Autodesk Inventor part; units mm, degrees
(part 7 of 8)
  arc A913 (19.6836, 30.4546) -> (19.6836, 30.4038) centre (19.6836, 30.4292) ccw
  arc A914 (19.9605, 30.3115) -> (19.991, 30.3522) centre (19.9757, 30.3318) ccw
  arc A915 (19.9757, 30.3318) -> (19.6836, 30.4292) centre (19.6836, 29.9424) ccw
  arc A916 (19.3986, 30.1696) -> (19.4494, 30.1696) centre (19.424, 30.1696) ccw
  arc A917 (19.6836, 30.4038) -> (19.6836, 30.4546) centre (19.6836, 30.4292) ccw
  arc A918 (19.6836, 30.4292) -> (19.424, 30.1696) centre (19.6836, 30.1696) ccw
  arc A919 (19.781, 29.2354) -> (19.781, 29.2862) centre (19.781, 29.2608) ccw
  arc A920 (19.4096, 29.441) -> (19.3735, 29.4052) centre (19.3916, 29.4231) ccw
  arc A921 (19.3915, 29.4231) -> (19.781, 29.2608) centre (19.781, 29.8093) ccw
  arc A922 (20.066, 29.5204) -> (20.0152, 29.5204) centre (20.0406, 29.5204) ccw
  arc A923 (19.781, 29.2862) -> (19.781, 29.2354) centre (19.781, 29.2608) ccw
  arc A924 (19.781, 29.2608) -> (20.0406, 29.5204) centre (19.781, 29.5204) ccw
  arc A925 (18.9204, 29.2494) -> (18.9658, 29.2722) centre (18.9431, 29.2608) ccw
  arc A926 (18.7062, 29.7914) -> (18.6607, 29.7687) centre (18.6835, 29.78) ccw
  line L282 (18.9431, 29.2608) -> (18.6835, 29.7801)
  arc A927 (18.6185, 29.7547) -> (18.6185, 29.8055) centre (18.6185, 29.7801) ccw
  arc A928 (18.294, 29.8055) -> (18.294, 29.7547) centre (18.294, 29.7801) ccw
  line L283 (18.6185, 29.7801) -> (18.294, 29.7801)
  arc A929 (18.6185, 30.4546) -> (18.6185, 30.4038) centre (18.6185, 30.4292) ccw
  arc A930 (18.6185, 29.8055) -> (18.6185, 29.7547) centre (18.6185, 29.7801) ccw
  arc A931 (18.6185, 29.7801) -> (18.6185, 30.4292) centre (18.6185, 30.1046) ccw
  arc A932 (18.294, 30.4546) -> (18.294, 30.4038) centre (18.294, 30.4292) ccw
  arc A933 (18.6185, 30.4038) -> (18.6185, 30.4546) centre (18.6185, 30.4292) ccw
  line L284 (18.294, 30.4292) -> (18.6185, 30.4292)
  arc A934 (18.2686, 29.2608) -> (18.3194, 29.2608) centre (18.294, 29.2608) ccw
  arc A935 (18.3194, 30.4292) -> (18.2686, 30.4292) centre (18.294, 30.4292) ccw
  line L285 (18.294, 29.2608) -> (18.294, 30.4292)
  arc A936 (17.78, 29.5854) -> (17.7292, 29.5854) centre (17.7546, 29.5854) ccw
  arc A937 (17.1309, 29.5854) -> (17.0801, 29.5854) centre (17.1055, 29.5854) ccw
  arc A938 (17.1055, 29.5854) -> (17.7546, 29.5854) centre (17.4301, 29.5854) ccw
  arc A939 (17.78, 30.1046) -> (17.7292, 30.1046) centre (17.7546, 30.1046) ccw
  arc A940 (17.7292, 29.5854) -> (17.78, 29.5854) centre (17.7546, 29.5854) ccw
  line L286 (17.7546, 30.1046) -> (17.7546, 29.5854)
  arc A941 (17.0801, 30.1046) -> (17.1309, 30.1046) centre (17.1055, 30.1046) ccw
  arc A942 (17.7292, 30.1046) -> (17.78, 30.1046) centre (17.7546, 30.1046) ccw
  arc A943 (17.7546, 30.1046) -> (17.1055, 30.1046) centre (17.4301, 30.1046) ccw
  arc A944 (17.0801, 29.5854) -> (17.1309, 29.5854) centre (17.1055, 29.5854) ccw
  arc A945 (17.1309, 30.1046) -> (17.0801, 30.1046) centre (17.1055, 30.1046) ccw
  line L287 (17.1055, 29.5854) -> (17.1055, 30.1046)
  arc A946 (16.5078, 29.7253) -> (16.5321, 29.7699) centre (16.5199, 29.7476) ccw
  arc A947 (16.1751, 29.9647) -> (16.1507, 29.9201) centre (16.1629, 29.9424) ccw
  line L288 (16.5199, 29.7476) -> (16.1629, 29.9424)
  arc A948 (16.5328, 29.7695) -> (16.507, 29.7257) centre (16.5199, 29.7476) ccw
  arc A949 (16.6243, 29.5204) -> (16.6751, 29.5204) centre (16.6497, 29.5204) ccw
  arc A950 (16.6497, 29.5204) -> (16.5199, 29.7476) centre (16.3861, 29.5204) ccw
  arc A951 (16.15, 29.9205) -> (16.1758, 29.9642) centre (16.1629, 29.9424) ccw
  arc A952 (16.0585, 30.1696) -> (16.0077, 30.1696) centre (16.0331, 30.1696) ccw
  arc A953 (16.0331, 30.1696) -> (16.1629, 29.9424) centre (16.2968, 30.1695) ccw
  arc A954 (16.2927, 30.4546) -> (16.2927, 30.4038) centre (16.2927, 30.4292) ccw
  arc A955 (16.5696, 30.3115) -> (16.6001, 30.3522) centre (16.5849, 30.3318) ccw
  arc A956 (16.5848, 30.3318) -> (16.2927, 30.4292) centre (16.2927, 29.9424) ccw
  arc A957 (16.0077, 30.1696) -> (16.0585, 30.1696) centre (16.0331, 30.1696) ccw
  arc A958 (16.2927, 30.4038) -> (16.2927, 30.4546) centre (16.2927, 30.4292) ccw
  arc A959 (16.2927, 30.4292) -> (16.0331, 30.1696) centre (16.2927, 30.1696) ccw
  arc A960 (16.3901, 29.2354) -> (16.3901, 29.2862) centre (16.3901, 29.2608) ccw
  arc A961 (16.0187, 29.441) -> (15.9826, 29.4052) centre (16.0007, 29.4231) ccw
  arc A962 (16.0006, 29.4231) -> (16.3901, 29.2608) centre (16.3901, 29.8093) ccw
  arc A963 (16.6751, 29.5204) -> (16.6243, 29.5204) centre (16.6497, 29.5204) ccw
  arc A964 (16.3901, 29.2862) -> (16.3901, 29.2354) centre (16.3901, 29.2608) ccw
  arc A965 (16.3901, 29.2608) -> (16.6497, 29.5204) centre (16.3901, 29.5204) ccw
  arc A966 (15.4813, 29.2608) -> (15.5321, 29.2608) centre (15.5067, 29.2608) ccw
  arc A967 (15.5321, 30.4292) -> (15.4813, 30.4292) centre (15.5067, 30.4292) ccw
  line L289 (15.5067, 29.2608) -> (15.5067, 30.4292)
  arc A968 (14.8798, 30.4415) -> (14.8354, 30.4169) centre (14.8576, 30.4292) ccw
  arc A969 (15.4845, 29.2485) -> (15.5289, 29.2731) centre (15.5067, 29.2608) ccw
  line L290 (14.8576, 30.4292) -> (15.5067, 29.2608)
  arc A970 (14.8322, 29.2608) -> (14.883, 29.2608) centre (14.8576, 29.2608) ccw
  arc A971 (14.883, 30.4292) -> (14.8322, 30.4292) centre (14.8576, 30.4292) ccw
  line L291 (14.8576, 29.2608) -> (14.8576, 30.4292)
  arc A972 (13.8693, 29.9353) -> (13.8693, 29.8845) centre (13.8693, 29.9099) ccw
  arc A973 (14.2588, 29.8845) -> (14.2588, 29.9353) centre (14.2588, 29.9099) ccw
  line L292 (13.8693, 29.9099) -> (14.2588, 29.9099)
  arc A974 (13.8693, 30.4546) -> (13.8693, 30.4038) centre (13.8693, 30.4292) ccw
  arc A975 (14.3886, 30.4038) -> (14.3886, 30.4546) centre (14.3886, 30.4292) ccw
  line L293 (13.8693, 30.4292) -> (14.3886, 30.4292)
  arc A976 (13.8439, 29.2608) -> (13.8947, 29.2608) centre (13.8693, 29.2608) ccw
  arc A977 (13.8947, 30.4292) -> (13.8439, 30.4292) centre (13.8693, 30.4292) ccw
  line L294 (13.8693, 29.2608) -> (13.8693, 30.4292)
  arc A978 (14.3886, 29.2354) -> (14.3886, 29.2862) centre (14.3886, 29.2608) ccw
  arc A979 (13.8693, 29.2862) -> (13.8693, 29.2354) centre (13.8693, 29.2608) ccw
  line L295 (14.3886, 29.2608) -> (13.8693, 29.2608)
  arc A980 (13.2312, 29.7253) -> (13.2555, 29.7699) centre (13.2433, 29.7476) ccw
  arc A981 (12.8985, 29.9647) -> (12.8741, 29.9201) centre (12.8863, 29.9424) ccw
  line L296 (13.2433, 29.7476) -> (12.8863, 29.9424)
  arc A982 (13.2562, 29.7695) -> (13.2304, 29.7257) centre (13.2433, 29.7476) ccw
  arc A983 (13.3477, 29.5204) -> (13.3985, 29.5204) centre (13.3731, 29.5204) ccw
  arc A984 (13.3731, 29.5204) -> (13.2433, 29.7476) centre (13.1095, 29.5204) ccw
  arc A985 (12.8734, 29.9205) -> (12.8992, 29.9642) centre (12.8863, 29.9424) ccw
  arc A986 (12.7819, 30.1696) -> (12.7311, 30.1696) centre (12.7565, 30.1696) ccw
  arc A987 (12.7565, 30.1696) -> (12.8863, 29.9424) centre (13.0202, 30.1695) ccw
  arc A988 (13.0161, 30.4546) -> (13.0161, 30.4038) centre (13.0161, 30.4292) ccw
  arc A989 (13.293, 30.3115) -> (13.3235, 30.3522) centre (13.3082, 30.3318) ccw
  arc A990 (13.3082, 30.3318) -> (13.0161, 30.4292) centre (13.0161, 29.9424) ccw
  arc A991 (12.7311, 30.1696) -> (12.7819, 30.1696) centre (12.7565, 30.1696) ccw
  arc A992 (13.0161, 30.4038) -> (13.0161, 30.4546) centre (13.0161, 30.4292) ccw
  arc A993 (13.0161, 30.4292) -> (12.7565, 30.1696) centre (13.0161, 30.1696) ccw
  arc A994 (13.1135, 29.2354) -> (13.1135, 29.2862) centre (13.1135, 29.2608) ccw
  arc A995 (12.7421, 29.441) -> (12.706, 29.4052) centre (12.7241, 29.4231) ccw
  arc A996 (12.724, 29.4231) -> (13.1135, 29.2608) centre (13.1135, 29.8093) ccw
  arc A997 (13.3985, 29.5204) -> (13.3477, 29.5204) centre (13.3731, 29.5204) ccw
  arc A998 (13.1135, 29.2862) -> (13.1135, 29.2354) centre (13.1135, 29.2608) ccw
  arc A999 (13.1135, 29.2608) -> (13.3731, 29.5204) centre (13.1135, 29.5204) ccw
  arc A1000 (83.7121, 29.1084) -> (83.801, 29.1084) centre (83.7565, 29.1084) ccw
  arc A1001 (83.801, 30.7086) -> (83.7121, 30.7086) centre (83.7566, 30.7086) ccw
  line L297 (83.7565, 29.1084) -> (83.7565, 30.7086)
  arc A1002 (82.9064, 30.7302) -> (82.8286, 30.687) centre (82.8675, 30.7086) ccw
  arc A1003 (83.7176, 29.0868) -> (83.7954, 29.13) centre (83.7565, 29.1084) ccw
  line L298 (82.8675, 30.7086) -> (83.7565, 29.1084)
  arc A1004 (82.8231, 29.1084) -> (82.912, 29.1084) centre (82.8675, 29.1084) ccw
  arc A1005 (82.912, 30.7086) -> (82.8231, 30.7086) centre (82.8676, 30.7086) ccw
  line L299 (82.8675, 29.1084) -> (82.8675, 30.7086)
  arc A1006 (81.8316, 30.7531) -> (81.8316, 30.6641) centre (81.8316, 30.7086) ccw
  arc A1007 (82.1872, 30.6641) -> (82.1872, 30.7531) centre (82.1872, 30.7086) ccw
  line L300 (81.8316, 30.7086) -> (82.1872, 30.7086)
  arc A1008 (81.8316, 29.1529) -> (81.8316, 29.064) centre (81.8316, 29.1085) ccw
  arc A1009 (82.1872, 29.064) -> (82.1872, 29.1529) centre (82.1872, 29.1085) ccw
  line L301 (81.8316, 29.1084) -> (82.1872, 29.1084)
  arc A1010 (82.0538, 30.7086) -> (81.965, 30.7086) centre (82.0094, 30.7086) ccw
  arc A1011 (81.965, 29.1084) -> (82.0538, 29.1084) centre (82.0094, 29.1084) ccw
  line L302 (82.0094, 30.7086) -> (82.0094, 29.1084)
  arc A1012 (80.5596, 28.9751) -> (80.5596, 28.8862) centre (80.5596, 28.9306) ccw
  arc A1013 (81.2708, 28.8862) -> (81.2708, 28.9751) centre (81.2708, 28.9306) ccw
  line L303 (80.5596, 28.9306) -> (81.2708, 28.9306)
  arc A1014 (79.9232, 29.0885) -> (80.0028, 29.1283) centre (79.963, 29.1084) ccw
  arc A1015 (79.6472, 29.8395) -> (79.5676, 29.7997) centre (79.6074, 29.8196) ccw
  line L304 (79.963, 29.1084) -> (79.6074, 29.8196)
  arc A1016 (79.5185, 29.7752) -> (79.5185, 29.8641) centre (79.5185, 29.8197) ccw
  arc A1017 (79.074, 29.8641) -> (79.074, 29.7752) centre (79.074, 29.8197) ccw
  line L305 (79.5185, 29.8196) -> (79.074, 29.8196)
  arc A1018 (79.5185, 30.7531) -> (79.5185, 30.6641) centre (79.5185, 30.7086) ccw
  arc A1019 (79.5185, 29.8641) -> (79.5185, 29.7752) centre (79.5185, 29.8197) ccw
  arc A1020 (79.5185, 29.8196) -> (79.5185, 30.7086) centre (79.5185, 30.2641) ccw
  arc A1021 (79.074, 30.7531) -> (79.074, 30.6641) centre (79.074, 30.7086) ccw
  arc A1022 (79.5185, 30.6641) -> (79.5185, 30.7531) centre (79.5185, 30.7086) ccw
  line L306 (79.074, 30.7086) -> (79.5185, 30.7086)
  arc A1023 (79.0295, 29.1084) -> (79.1184, 29.1084) centre (79.0739, 29.1084) ccw
  arc A1024 (79.1184, 30.7086) -> (79.0295, 30.7086) centre (79.0739, 30.7086) ccw
  line L307 (79.074, 29.1084) -> (79.074, 30.7086)
  arc A1025 (77.7125, 30.0419) -> (77.7125, 29.953) centre (77.7125, 29.9975) ccw
  arc A1026 (78.2459, 29.953) -> (78.2459, 30.0419) centre (78.2459, 29.9975) ccw
  line L308 (77.7125, 29.9974) -> (78.2459, 29.9974)
  arc A1027 (77.7125, 30.7531) -> (77.7125, 30.6641) centre (77.7125, 30.7086) ccw
  arc A1028 (78.4237, 30.6641) -> (78.4237, 30.7531) centre (78.4237, 30.7086) ccw
  line L309 (77.7125, 30.7086) -> (78.4237, 30.7086)
  arc A1029 (77.668, 29.1084) -> (77.7569, 29.1084) centre (77.7125, 29.1084) ccw
  arc A1030 (77.7569, 30.7086) -> (77.668, 30.7086) centre (77.7125, 30.7086) ccw
  line L310 (77.7125, 29.1084) -> (77.7125, 30.7086)
  arc A1031 (78.4237, 29.064) -> (78.4237, 29.1529) centre (78.4237, 29.1085) ccw
  arc A1032 (77.7125, 29.1529) -> (77.7125, 29.064) centre (77.7125, 29.1085) ccw
  line L311 (78.4237, 29.1084) -> (77.7125, 29.1084)
  arc A1033 (76.6423, 29.118) -> (76.7291, 29.0988) centre (76.6857, 29.1084) ccw
  arc A1034 (77.0847, 30.699) -> (76.9979, 30.7182) centre (77.0413, 30.7086) ccw
  line L312 (76.6857, 29.1084) -> (77.0413, 30.7086)
  arc A1035 (76.3722, 30.1893) -> (76.2879, 30.1611) centre (76.33, 30.1752) ccw
  arc A1036 (76.6435, 29.0943) -> (76.7278, 29.1225) centre (76.6857, 29.1084) ccw
  line L313 (76.3301, 30.1752) -> (76.6857, 29.1084)
  arc A1037 (75.9323, 29.1225) -> (76.0166, 29.0943) centre (75.9744, 29.1084) ccw
  arc A1038 (76.3722, 30.1611) -> (76.2879, 30.1893) centre (76.33, 30.1752) ccw
  line L314 (75.9745, 29.1084) -> (76.3301, 30.1752)
  arc A1039 (75.6623, 30.7182) -> (75.5755, 30.699) centre (75.6189, 30.7086) ccw
  arc A1040 (75.9311, 29.0988) -> (76.0179, 29.118) centre (75.9745, 29.1084) ccw
  line L315 (75.6189, 30.7086) -> (75.9745, 29.1084)
  arc A1041 (75.0475, 29.5529) -> (74.9586, 29.5529) centre (75.0031, 29.5529) ccw
  arc A1042 (74.1585, 29.5529) -> (74.0696, 29.5529) centre (74.114, 29.5529) ccw
  arc A1043 (74.114, 29.5529) -> (75.003, 29.5529) centre (74.5585, 29.5529) ccw
  arc A1044 (75.0475, 30.2641) -> (74.9586, 30.2641) centre (75.0031, 30.2641) ccw
  arc A1045 (74.9586, 29.5529) -> (75.0475, 29.5529) centre (75.0031, 29.5529) ccw
  line L316 (75.003, 30.2641) -> (75.003, 29.5529)
  arc A1046 (74.0696, 30.2641) -> (74.1585, 30.2641) centre (74.114, 30.2641) ccw
  arc A1047 (74.9586, 30.2641) -> (75.0475, 30.2641) centre (75.0031, 30.2641) ccw
  arc A1048 (75.003, 30.2641) -> (74.114, 30.2641) centre (74.5585, 30.2641) ccw
  arc A1049 (74.0696, 29.5529) -> (74.1585, 29.5529) centre (74.114, 29.5529) ccw
  arc A1050 (74.1585, 30.2641) -> (74.0696, 30.2641) centre (74.114, 30.2641) ccw
  line L317 (74.114, 29.5529) -> (74.114, 30.2641)
  arc A1051 (73.0707, 29.7752) -> (73.0707, 29.8641) centre (73.0707, 29.8197) ccw
  arc A1052 (72.6262, 29.8641) -> (72.6262, 29.7752) centre (72.6262, 29.8197) ccw
  line L318 (73.0707, 29.8196) -> (72.6262, 29.8196)
  arc A1053 (73.0707, 30.7531) -> (73.0707, 30.6641) centre (73.0707, 30.7086) ccw
  arc A1054 (73.0707, 29.8641) -> (73.0707, 29.7752) centre (73.0707, 29.8197) ccw
  arc A1055 (73.0707, 29.8196) -> (73.0707, 30.7086) centre (73.0707, 30.2641) ccw
  arc A1056 (72.6262, 30.7531) -> (72.6262, 30.6641) centre (72.6262, 30.7086) ccw
  arc A1057 (73.0707, 30.6641) -> (73.0707, 30.7531) centre (73.0707, 30.7086) ccw
  line L319 (72.6262, 30.7086) -> (73.0707, 30.7086)
  arc A1058 (72.5818, 29.1084) -> (72.6707, 29.1084) centre (72.6262, 29.1084) ccw
  arc A1059 (72.6707, 30.7086) -> (72.5818, 30.7086) centre (72.6262, 30.7086) ccw
  line L320 (72.6262, 29.1084) -> (72.6262, 30.7086)
  arc A1060 (59.8236, 29.7253) -> (59.8479, 29.7699) centre (59.8358, 29.7476) ccw
  arc A1061 (59.4909, 29.9647) -> (59.4666, 29.9201) centre (59.4788, 29.9424) ccw
  line L321 (59.8358, 29.7476) -> (59.4788, 29.9424)
  arc A1062 (59.8487, 29.7695) -> (59.8229, 29.7257) centre (59.8358, 29.7476) ccw
  arc A1063 (59.9402, 29.5204) -> (59.991, 29.5204) centre (59.9656, 29.5204) ccw
  arc A1064 (59.9656, 29.5204) -> (59.8358, 29.7476) centre (59.7019, 29.5204) ccw
  arc A1065 (59.4659, 29.9205) -> (59.4916, 29.9642) centre (59.4787, 29.9424) ccw
  arc A1066 (59.3743, 30.1696) -> (59.3235, 30.1696) centre (59.3489, 30.1696) ccw
  arc A1067 (59.3489, 30.1696) -> (59.4788, 29.9424) centre (59.6126, 30.1696) ccw
  arc A1068 (59.6086, 30.4546) -> (59.6086, 30.4038) centre (59.6086, 30.4292) ccw
  arc A1069 (59.8855, 30.3115) -> (59.9159, 30.3522) centre (59.9007, 30.3318) ccw
  arc A1070 (59.9007, 30.3318) -> (59.6086, 30.4292) centre (59.6086, 29.9424) ccw
  arc A1071 (59.3235, 30.1696) -> (59.3743, 30.1696) centre (59.3489, 30.1696) ccw
  arc A1072 (59.6086, 30.4038) -> (59.6086, 30.4546) centre (59.6086, 30.4292) ccw
  arc A1073 (59.6086, 30.4292) -> (59.3489, 30.1696) centre (59.6086, 30.1695) ccw
  arc A1074 (59.706, 29.2354) -> (59.706, 29.2862) centre (59.706, 29.2608) ccw
  arc A1075 (59.3345, 29.441) -> (59.2985, 29.4052) centre (59.3165, 29.4231) ccw
  arc A1076 (59.3165, 29.4231) -> (59.706, 29.2608) centre (59.706, 29.8094) ccw
  arc A1077 (59.991, 29.5204) -> (59.9402, 29.5204) centre (59.9656, 29.5204) ccw
  arc A1078 (59.706, 29.2862) -> (59.706, 29.2354) centre (59.706, 29.2608) ccw
  arc A1079 (59.706, 29.2608) -> (59.9656, 29.5204) centre (59.706, 29.5204) ccw
  arc A1080 (58.8453, 29.2494) -> (58.8908, 29.2722) centre (58.868, 29.2608) ccw
  arc A1081 (58.6311, 29.7914) -> (58.5857, 29.7687) centre (58.6084, 29.78) ccw
  line L322 (58.8681, 29.2608) -> (58.6084, 29.7801)
  arc A1082 (58.5435, 29.7547) -> (58.5435, 29.8055) centre (58.5435, 29.7801) ccw
  arc A1083 (58.219, 29.8055) -> (58.219, 29.7547) centre (58.219, 29.7801) ccw
  line L323 (58.5435, 29.7801) -> (58.219, 29.7801)
  arc A1084 (58.5435, 30.4546) -> (58.5435, 30.4038) centre (58.5435, 30.4292) ccw
  arc A1085 (58.5435, 29.8055) -> (58.5435, 29.7547) centre (58.5435, 29.7801) ccw
  arc A1086 (58.5435, 29.7801) -> (58.5435, 30.4292) centre (58.5435, 30.1046) ccw
  arc A1087 (58.5435, 30.4038) -> (58.5435, 30.4546) centre (58.5435, 30.4292) ccw
  line L324 (58.219, 30.4292) -> (58.5435, 30.4292)
  arc A1088 (58.1936, 29.2608) -> (58.2444, 29.2608) centre (58.219, 29.2608) ccw
  arc A1089 (58.2444, 30.4292) -> (58.1936, 30.4292) centre (58.219, 30.4292) ccw
  line L325 (58.219, 29.2608) -> (58.219, 30.4292)
  arc A1090 (57.705, 29.5854) -> (57.6542, 29.5854) centre (57.6796, 29.5854) ccw
  arc A1091 (57.0559, 29.5854) -> (57.0051, 29.5854) centre (57.0305, 29.5854) ccw
  arc A1092 (57.0305, 29.5854) -> (57.6796, 29.5854) centre (57.3551, 29.5854) ccw
  arc A1093 (57.705, 30.1046) -> (57.6542, 30.1046) centre (57.6796, 30.1046) ccw
  arc A1094 (57.6542, 29.5854) -> (57.705, 29.5854) centre (57.6796, 29.5854) ccw
  line L326 (57.6796, 30.1046) -> (57.6796, 29.5854)
  arc A1095 (57.0051, 30.1046) -> (57.0559, 30.1046) centre (57.0305, 30.1046) ccw
  arc A1096 (57.6542, 30.1046) -> (57.705, 30.1046) centre (57.6796, 30.1046) ccw
  arc A1097 (57.6796, 30.1046) -> (57.0305, 30.1046) centre (57.3551, 30.1046) ccw
  arc A1098 (57.0051, 29.5854) -> (57.0559, 29.5854) centre (57.0305, 29.5854) ccw
  arc A1099 (57.0559, 30.1046) -> (57.0051, 30.1046) centre (57.0305, 30.1046) ccw
  line L327 (57.0305, 29.5854) -> (57.0305, 30.1046)
  arc A1100 (55.9637, 30.4546) -> (55.9637, 30.4038) centre (55.9637, 30.4292) ccw
  arc A1101 (56.6128, 30.4038) -> (56.6128, 30.4546) centre (56.6128, 30.4292) ccw
  line L328 (55.9637, 30.4292) -> (56.6128, 30.4292)
  arc A1102 (56.2629, 29.2608) -> (56.3137, 29.2608) centre (56.2883, 29.2608) ccw
  arc A1103 (56.3137, 30.4292) -> (56.2629, 30.4292) centre (56.2883, 30.4292) ccw
  line L329 (56.2883, 29.2608) -> (56.2883, 30.4292)
  arc A1104 (55.5714, 29.5854) -> (55.5206, 29.5854) centre (55.546, 29.5854) ccw
  arc A1105 (54.9223, 29.5854) -> (54.8715, 29.5854) centre (54.8969, 29.5854) ccw
  arc A1106 (54.8969, 29.5854) -> (55.546, 29.5854) centre (55.2215, 29.5854) ccw
  arc A1107 (55.5714, 30.1046) -> (55.5206, 30.1046) centre (55.546, 30.1046) ccw
  arc A1108 (55.5206, 29.5854) -> (55.5714, 29.5854) centre (55.546, 29.5854) ccw
  line L330 (55.546, 30.1046) -> (55.546, 29.5854)
  arc A1109 (54.8715, 30.1046) -> (54.9223, 30.1046) centre (54.8969, 30.1046) ccw
  arc A1110 (55.5206, 30.1046) -> (55.5714, 30.1046) centre (55.546, 30.1046) ccw
  arc A1111 (55.546, 30.1046) -> (54.8969, 30.1046) centre (55.2215, 30.1046) ccw
  arc A1112 (54.8715, 29.5854) -> (54.9223, 29.5854) centre (54.8969, 29.5854) ccw
  arc A1113 (54.9223, 30.1046) -> (54.8715, 30.1046) centre (54.8969, 30.1046) ccw
  line L331 (54.8969, 29.5854) -> (54.8969, 30.1046)
  arc A1114 (54.379, 30.4292) -> (54.3282, 30.4292) centre (54.3536, 30.4292) ccw
  arc A1115 (54.3282, 29.2608) -> (54.379, 29.2608) centre (54.3536, 29.2608) ccw
  line L332 (54.3536, 30.4292) -> (54.3536, 29.2608)
  arc A1116 (53.9424, 29.7932) -> (53.9859, 29.767) centre (53.9642, 29.7801) ccw
  arc A1117 (54.3754, 30.4161) -> (54.3318, 30.4423) centre (54.3536, 30.4292) ccw
  line L333 (53.9642, 29.7801) -> (54.3536, 30.4292)
  arc A1118 (53.5965, 30.4423) -> (53.5529, 30.4161) centre (53.5747, 30.4292) ccw
  arc A1119 (53.9424, 29.767) -> (53.9859, 29.7932) centre (53.9642, 29.7801) ccw
  line L334 (53.5747, 30.4292) -> (53.9642, 29.7801)
  arc A1120 (53.5493, 29.2608) -> (53.6001, 29.2608) centre (53.5747, 29.2608) ccw
  arc A1121 (53.6001, 30.4292) -> (53.5493, 30.4292) centre (53.5747, 30.4292) ccw
  line L335 (53.5747, 29.2608) -> (53.5747, 30.4292)
  arc A1122 (43.4332, 22.9743) -> (43.4332, 22.8981) centre (43.4332, 22.9362) ccw
  arc A1123 (44.3363, 22.8981) -> (44.3363, 22.9743) centre (44.3363, 22.9362) ccw
  line L336 (43.4332, 22.9362) -> (44.3363, 22.9362)
  arc A1124 (43.9228, 24.5618) -> (43.8466, 24.5618) centre (43.8847, 24.5618) ccw
  arc A1125 (43.8466, 22.9362) -> (43.9228, 22.9362) centre (43.8847, 22.9362) ccw
  line L337 (43.8847, 24.5618) -> (43.8847, 22.9362)
  arc A1126 (43.4094, 24.2303) -> (43.457, 24.1708) centre (43.4332, 24.2005) ccw
  arc A1127 (43.9085, 24.532) -> (43.8609, 24.5916) centre (43.8847, 24.5618) ccw
  line L338 (43.4332, 24.2006) -> (43.8847, 24.5618)
  arc A1128 (41.8701, 22.9743) -> (41.8701, 22.8981) centre (41.8701, 22.9362) ccw
  arc A1129 (42.7732, 22.8981) -> (42.7732, 22.9743) centre (42.7732, 22.9362) ccw
  line L339 (41.8701, 22.9362) -> (42.7732, 22.9362)
  arc A1130 (42.6667, 23.8146) -> (42.6087, 23.864) centre (42.6377, 23.8393) ccw
  arc A1131 (41.841, 22.9609) -> (41.8991, 22.9115) centre (41.87, 22.9362) ccw
  line L340 (42.6377, 23.8393) -> (41.8701, 22.9362)
  arc A1132 (42.8113, 24.1554) -> (42.7351, 24.1554) centre (42.7732, 24.1554) ccw
  arc A1133 (42.6114, 23.8669) -> (42.664, 23.8117) centre (42.6377, 23.8393) ccw
  arc A1134 (42.6377, 23.8393) -> (42.7732, 24.1554) centre (42.3367, 24.1554) ccw
  arc A1135 (41.8338, 24.2123) -> (41.9063, 24.1888) centre (41.87, 24.2005) ccw
  arc A1136 (42.3668, 24.5237) -> (42.3668, 24.5999) centre (42.3668, 24.5618) ccw
  arc A1137 (42.3668, 24.5618) -> (41.8701, 24.2006) centre (42.3668, 24.0397) ccw
  arc A1138 (42.3668, 24.5999) -> (42.3668, 24.5237) centre (42.3668, 24.5618) ccw
  arc A1139 (42.7351, 24.1554) -> (42.8113, 24.1554) centre (42.7732, 24.1554) ccw
  arc A1140 (42.7732, 24.1554) -> (42.3668, 24.5618) centre (42.3668, 24.1554) ccw
  arc A1141 (40.3675, 23.3212) -> (40.427, 23.2736) centre (40.3972, 23.2974) ccw
  arc A1142 (41.1495, 24.1768) -> (41.09, 24.2244) centre (41.1198, 24.2006) ccw
  line L341 (40.3973, 23.2974) -> (41.1197, 24.2006)
  arc A1143 (41.1106, 23.1496) -> (41.0386, 23.1743) centre (41.0746, 23.162) ccw
  arc A1144 (40.7585, 22.9743) -> (40.7585, 22.8981) centre (40.7585, 22.9362) ccw
  arc A1145 (40.7585, 22.9362) -> (41.0746, 23.162) centre (40.7585, 23.2703) ccw
  arc A1146 (41.2482, 23.749) -> (41.172, 23.749) centre (41.2101, 23.749) ccw
  arc A1147 (41.0403, 23.1787) -> (41.1088, 23.1453) centre (41.0746, 23.162) ccw
  arc A1148 (41.0746, 23.162) -> (41.2101, 23.749) centre (39.8707, 23.7491) ccw
  arc A1149 (40.7585, 22.8981) -> (40.7585, 22.9743) centre (40.7585, 22.9362) ccw
  arc A1150 (40.4785, 23.1743) -> (40.4064, 23.1496) centre (40.4424, 23.162) ccw
  arc A1151 (40.4424, 23.162) -> (40.7585, 22.9362) centre (40.7585, 23.2703) ccw
  arc A1152 (40.4082, 23.1453) -> (40.4767, 23.1787) centre (40.4425, 23.162) ccw
  arc A1153 (40.345, 23.749) -> (40.2688, 23.749) centre (40.3069, 23.749) ccw
  arc A1154 (40.3069, 23.749) -> (40.4424, 23.162) centre (41.6463, 23.7491) ccw
  arc A1155 (41.1088, 24.3527) -> (41.0403, 24.3193) centre (41.0746, 24.336) ccw
  arc A1156 (41.172, 23.749) -> (41.2482, 23.749) centre (41.2101, 23.749) ccw
  arc A1157 (41.2101, 23.749) -> (41.0746, 24.336) centre (39.8707, 23.7489) ccw
  arc A1158 (40.7585, 24.5999) -> (40.7585, 24.5237) centre (40.7585, 24.5618) ccw
  arc A1159 (41.0386, 24.3237) -> (41.1106, 24.3484) centre (41.0746, 24.3361) ccw
  arc A1160 (41.0746, 24.336) -> (40.7585, 24.5618) centre (40.7585, 24.2277) ccw
  arc A1161 (40.4064, 24.3484) -> (40.4785, 24.3237) centre (40.4424, 24.3361) ccw
  arc A1162 (40.7585, 24.5237) -> (40.7585, 24.5999) centre (40.7585, 24.5618) ccw
  arc A1163 (40.7585, 24.5618) -> (40.4424, 24.336) centre (40.7585, 24.2277) ccw
  arc A1164 (40.2688, 23.749) -> (40.345, 23.749) centre (40.3069, 23.749) ccw
  arc A1165 (40.4767, 24.3193) -> (40.4082, 24.3527) centre (40.4425, 24.336) ccw
  arc A1166 (40.4424, 24.336) -> (40.3069, 23.749) centre (41.6463, 23.7489) ccw
  arc A1167 (38.7438, 22.9743) -> (38.7438, 22.8981) centre (38.7438, 22.9362) ccw
  arc A1168 (39.6469, 22.8981) -> (39.6469, 22.9743) centre (39.6469, 22.9362) ccw
  line L342 (38.7438, 22.9362) -> (39.6469, 22.9362)
  arc A1169 (39.5405, 23.8146) -> (39.4824, 23.864) centre (39.5114, 23.8393) ccw
  arc A1170 (38.7148, 22.9609) -> (38.7729, 22.9115) centre (38.7438, 22.9362) ccw
  line L343 (39.5115, 23.8393) -> (38.7438, 22.9362)
  arc A1171 (39.685, 24.1554) -> (39.6088, 24.1554) centre (39.6469, 24.1554) ccw
  arc A1172 (39.4852, 23.8669) -> (39.5377, 23.8117) centre (39.5114, 23.8393) ccw
  arc A1173 (39.5115, 23.8393) -> (39.6469, 24.1554) centre (39.2105, 24.1553) ccw
  arc A1174 (38.7076, 24.2123) -> (38.7801, 24.1888) centre (38.7438, 24.2005) ccw
  arc A1175 (39.2405, 24.5237) -> (39.2405, 24.5999) centre (39.2405, 24.5618) ccw
  arc A1176 (39.2405, 24.5618) -> (38.7438, 24.2006) centre (39.2405, 24.0397) ccw
  arc A1177 (39.2405, 24.5999) -> (39.2405, 24.5237) centre (39.2405, 24.5618) ccw
  arc A1178 (39.6088, 24.1554) -> (39.685, 24.1554) centre (39.6469, 24.1554) ccw
  arc A1179 (39.6469, 24.1554) -> (39.2405, 24.5618) centre (39.2405, 24.1554) ccw
  arc A1180 (36.1525, 23.6065) -> (36.1525, 23.5303) centre (36.1525, 23.5684) ccw
  arc A1181 (37.2363, 23.5303) -> (37.2363, 23.6065) centre (37.2363, 23.5684) ccw
  line L344 (36.1525, 23.5684) -> (37.2363, 23.5684)
  arc A1182 (34.0053, 22.9743) -> (34.0053, 22.8981) centre (34.0053, 22.9362) ccw
  arc A1183 (34.7278, 22.8981) -> (34.7278, 22.9743) centre (34.7278, 22.9362) ccw
  line L345 (34.0053, 22.9362) -> (34.7278, 22.9362)
  arc A1184 (34.0434, 24.5618) -> (33.9672, 24.5618) centre (34.0053, 24.5618) ccw
  arc A1185 (33.9672, 22.9362) -> (34.0434, 22.9362) centre (34.0053, 22.9362) ccw
  line L346 (34.0053, 24.5618) -> (34.0053, 22.9362)
  arc A1186 (33.3283, 23.3878) -> (33.2521, 23.3878) centre (33.2902, 23.3878) ccw
  arc A1187 (32.4252, 23.3878) -> (32.349, 23.3878) centre (32.3871, 23.3878) ccw
  arc A1188 (32.3871, 23.3878) -> (33.2902, 23.3878) centre (32.8387, 23.3878) ccw
  arc A1189 (33.3283, 24.1102) -> (33.2521, 24.1102) centre (33.2902, 24.1102) ccw
  arc A1190 (33.2521, 23.3878) -> (33.3283, 23.3878) centre (33.2902, 23.3878) ccw
  line L347 (33.2902, 24.1102) -> (33.2902, 23.3878)
  arc A1191 (32.349, 24.1102) -> (32.4252, 24.1102) centre (32.3871, 24.1102) ccw
  arc A1192 (33.2521, 24.1102) -> (33.3283, 24.1102) centre (33.2902, 24.1102) ccw
  arc A1193 (33.2902, 24.1102) -> (32.3871, 24.1102) centre (32.8387, 24.1102) ccw
  arc A1194 (32.349, 23.3878) -> (32.4252, 23.3878) centre (32.3871, 23.3878) ccw
  arc A1195 (32.4252, 24.1102) -> (32.349, 24.1102) centre (32.3871, 24.1102) ccw
  line L348 (32.3871, 23.3878) -> (32.3871, 24.1102)
  arc A1196 (31.4418, 24.5999) -> (31.4418, 24.5237) centre (31.4418, 24.5618) ccw
  arc A1197 (31.8031, 24.5237) -> (31.8031, 24.5999) centre (31.8031, 24.5618) ccw
  line L349 (31.4418, 24.5618) -> (31.8031, 24.5618)
  arc A1198 (31.0425, 24.2006) -> (31.1187, 24.2006) centre (31.0806, 24.2006) ccw
  arc A1199 (31.4418, 24.5237) -> (31.4418, 24.5999) centre (31.4418, 24.5618) ccw
  arc A1200 (31.4418, 24.5618) -> (31.0806, 24.2006) centre (31.4418, 24.2006) ccw
  arc A1201 (31.0425, 23.2974) -> (31.1187, 23.2974) centre (31.0806, 23.2974) ccw
  arc A1202 (31.1187, 24.2006) -> (31.0425, 24.2006) centre (31.0806, 24.2006) ccw
  line L350 (31.0806, 23.2974) -> (31.0806, 24.2006)
  arc A1203 (31.4418, 22.8981) -> (31.4418, 22.9743) centre (31.4418, 22.9362) ccw
  arc A1204 (31.1187, 23.2974) -> (31.0425, 23.2974) centre (31.0806, 23.2974) ccw
  arc A1205 (31.0806, 23.2974) -> (31.4418, 22.9362) centre (31.4418, 23.2974) ccw
  arc A1206 (31.8031, 22.8981) -> (31.8031, 22.9743) centre (31.8031, 22.9362) ccw
  arc A1207 (31.4418, 22.9743) -> (31.4418, 22.8981) centre (31.4418, 22.9362) ccw
  line L351 (31.8031, 22.9362) -> (31.4418, 22.9362)
  arc A1208 (30.4626, 23.3878) -> (30.3864, 23.3878) centre (30.4245, 23.3878) ccw
  arc A1209 (29.5595, 23.3878) -> (29.4833, 23.3878) centre (29.5214, 23.3878) ccw
  arc A1210 (29.5214, 23.3878) -> (30.4245, 23.3878) centre (29.9729, 23.3878) ccw
  arc A1211 (30.4626, 24.1102) -> (30.3864, 24.1102) centre (30.4245, 24.1102) ccw
  arc A1212 (30.3864, 23.3878) -> (30.4626, 23.3878) centre (30.4245, 23.3878) ccw
  line L352 (30.4245, 24.1102) -> (30.4245, 23.3878)
  constraints: 2604 point on circle, 1213 centre point, 704 end point, 233 point on line, 15 midpoint, 10 other
sketch "51" plane through (0, 0, 0) normal (0, 0, 1) x (1, 0, 0)
  arc A0 (23.1521, 24.892) -> (23.0759, 24.892) centre (23.114, 24.892) ccw
  arc A1 (23.0759, 24.638) -> (23.1521, 24.638) centre (23.114, 24.638) ccw
  line L0 (23.114, 24.892) -> (23.368, 24.892)
  arc A2 (23.368, 24.8539) -> (23.368, 24.9301) centre (23.368, 24.892) ccw
  arc A3 (23.114, 24.9301) -> (23.114, 24.8539) centre (23.114, 24.892) ccw
  line L1 (23.368, 24.892) -> (23.368, 25.908)
  arc A4 (23.4061, 25.908) -> (23.3299, 25.908) centre (23.368, 25.908) ccw
  arc A5 (23.3299, 24.892) -> (23.4061, 24.892) centre (23.368, 24.892) ccw
  line L2 (23.368, 25.908) -> (23.114, 25.908)
  line L3 (10.414, 24.638) -> (10.414, 24.892)
  arc A6 (10.4521, 24.892) -> (10.3759, 24.892) centre (10.414, 24.892) ccw
  arc A7 (10.3759, 24.638) -> (10.4521, 24.638) centre (10.414, 24.638) ccw
  line L4 (10.414, 24.892) -> (10.668, 24.892)
  arc A8 (10.668, 24.8539) -> (10.668, 24.9301) centre (10.668, 24.892) ccw
  arc A9 (10.414, 24.9301) -> (10.414, 24.8539) centre (10.414, 24.892) ccw
  line L5 (10.668, 24.892) -> (10.668, 25.908)
  arc A10 (10.7061, 25.908) -> (10.6299, 25.908) centre (10.668, 25.908) ccw
  arc A11 (10.6299, 24.892) -> (10.7061, 24.892) centre (10.668, 24.892) ccw
  line L6 (10.668, 25.908) -> (10.414, 25.908)
  arc A12 (10.414, 25.9461) -> (10.414, 25.8699) centre (10.414, 25.908) ccw
  arc A13 (10.668, 25.8699) -> (10.668, 25.9461) centre (10.668, 25.908) ccw
  line L7 (10.414, 25.908) -> (10.414, 26.162)
  arc A14 (10.4521, 26.162) -> (10.3759, 26.162) centre (10.414, 26.162) ccw
  arc A15 (10.3759, 25.908) -> (10.4521, 25.908) centre (10.414, 25.908) ccw
  line L8 (10.414, 26.162) -> (9.906, 26.162)
  arc A16 (9.906, 26.2001) -> (9.906, 26.1239) centre (9.906, 26.162) ccw
  arc A17 (10.414, 26.1239) -> (10.414, 26.2001) centre (10.414, 26.162) ccw
  line L9 (9.906, 26.162) -> (9.906, 25.908)
  arc A18 (9.8679, 25.908) -> (9.9441, 25.908) centre (9.906, 25.908) ccw
  arc A19 (9.9441, 26.162) -> (9.8679, 26.162) centre (9.906, 26.162) ccw
  line L10 (9.906, 25.908) -> (9.652, 25.908)
  arc A20 (9.652, 25.9461) -> (9.652, 25.8699) centre (9.652, 25.908) ccw
  arc A21 (9.906, 25.8699) -> (9.906, 25.9461) centre (9.906, 25.908) ccw
  line L11 (9.652, 25.908) -> (9.652, 24.892)
  arc A22 (9.6139, 24.892) -> (9.6901, 24.892) centre (9.652, 24.892) ccw
  arc A23 (9.6901, 25.908) -> (9.6139, 25.908) centre (9.652, 25.908) ccw
  line L12 (9.652, 24.892) -> (9.906, 24.892)
  arc A24 (9.906, 24.8539) -> (9.906, 24.9301) centre (9.906, 24.892) ccw
  arc A25 (9.652, 24.9301) -> (9.652, 24.8539) centre (9.652, 24.892) ccw
  line L13 (9.906, 24.892) -> (9.906, 24.638)
  arc A26 (9.8679, 24.638) -> (9.9441, 24.638) centre (9.906, 24.638) ccw
  arc A27 (9.9441, 24.892) -> (9.8679, 24.892) centre (9.906, 24.892) ccw
  line L14 (9.906, 24.638) -> (10.414, 24.638)
  arc A28 (10.414, 24.5999) -> (10.414, 24.6761) centre (10.414, 24.638) ccw
  arc A29 (9.906, 24.6761) -> (9.906, 24.5999) centre (9.906, 24.638) ccw
  line L15 (7.874, 24.638) -> (7.874, 24.892)
  arc A30 (7.9121, 24.892) -> (7.8359, 24.892) centre (7.874, 24.892) ccw
  arc A31 (7.8359, 24.638) -> (7.9121, 24.638) centre (7.874, 24.638) ccw
  line L16 (7.874, 24.892) -> (8.128, 24.892)
  arc A32 (8.128, 24.8539) -> (8.128, 24.9301) centre (8.128, 24.892) ccw
  arc A33 (7.874, 24.9301) -> (7.874, 24.8539) centre (7.874, 24.892) ccw
  line L17 (8.128, 24.892) -> (8.128, 25.908)
  arc A34 (8.1661, 25.908) -> (8.0899, 25.908) centre (8.128, 25.908) ccw
  arc A35 (8.0899, 24.892) -> (8.1661, 24.892) centre (8.128, 24.892) ccw
  line L18 (8.128, 25.908) -> (7.874, 25.908)
  arc A36 (7.874, 25.9461) -> (7.874, 25.8699) centre (7.874, 25.908) ccw
  arc A37 (8.128, 25.8699) -> (8.128, 25.9461) centre (8.128, 25.908) ccw
  line L19 (7.874, 25.908) -> (7.874, 26.162)
  arc A38 (7.9121, 26.162) -> (7.8359, 26.162) centre (7.874, 26.162) ccw
  arc A39 (7.8359, 25.908) -> (7.9121, 25.908) centre (7.874, 25.908) ccw
  line L20 (7.874, 26.162) -> (7.366, 26.162)
  arc A40 (7.366, 26.2001) -> (7.366, 26.1239) centre (7.366, 26.162) ccw
  arc A41 (7.874, 26.1239) -> (7.874, 26.2001) centre (7.874, 26.162) ccw
  line L21 (7.366, 26.162) -> (7.366, 25.908)
  arc A42 (7.3279, 25.908) -> (7.4041, 25.908) centre (7.366, 25.908) ccw
  arc A43 (7.4041, 26.162) -> (7.3279, 26.162) centre (7.366, 26.162) ccw
  line L22 (7.366, 25.908) -> (7.112, 25.908)
  arc A44 (7.112, 25.9461) -> (7.112, 25.8699) centre (7.112, 25.908) ccw
  arc A45 (7.366, 25.8699) -> (7.366, 25.9461) centre (7.366, 25.908) ccw
  line L23 (7.112, 25.908) -> (7.112, 24.892)
  arc A46 (7.0739, 24.892) -> (7.1501, 24.892) centre (7.112, 24.892) ccw
  arc A47 (7.1501, 25.908) -> (7.0739, 25.908) centre (7.112, 25.908) ccw
  line L24 (7.112, 24.892) -> (7.366, 24.892)
  arc A48 (7.366, 24.8539) -> (7.366, 24.9301) centre (7.366, 24.892) ccw
  arc A49 (7.112, 24.9301) -> (7.112, 24.8539) centre (7.112, 24.892) ccw
  line L25 (7.366, 24.892) -> (7.366, 24.638)
  arc A50 (7.3279, 24.638) -> (7.4041, 24.638) centre (7.366, 24.638) ccw
  arc A51 (7.4041, 24.892) -> (7.3279, 24.892) centre (7.366, 24.892) ccw
  line L26 (7.366, 24.638) -> (7.874, 24.638)
  arc A52 (7.874, 24.5999) -> (7.874, 24.6761) centre (7.874, 24.638) ccw
  arc A53 (7.366, 24.6761) -> (7.366, 24.5999) centre (7.366, 24.638) ccw
  arc A54 (23.114, 25.9461) -> (23.114, 25.8699) centre (23.114, 25.908) ccw
  arc A55 (23.368, 25.8699) -> (23.368, 25.9461) centre (23.368, 25.908) ccw
  line L27 (23.114, 25.908) -> (23.114, 26.162)
  arc A56 (23.1521, 26.162) -> (23.0759, 26.162) centre (23.114, 26.162) ccw
  arc A57 (23.0759, 25.908) -> (23.1521, 25.908) centre (23.114, 25.908) ccw
  line L28 (23.114, 26.162) -> (22.606, 26.162)
  arc A58 (22.606, 26.2001) -> (22.606, 26.1239) centre (22.606, 26.162) ccw
  arc A59 (23.114, 26.1239) -> (23.114, 26.2001) centre (23.114, 26.162) ccw
  line L29 (22.606, 26.162) -> (22.606, 25.908)
  arc A60 (22.5679, 25.908) -> (22.6441, 25.908) centre (22.606, 25.908) ccw
  arc A61 (22.6441, 26.162) -> (22.5679, 26.162) centre (22.606, 26.162) ccw
  line L30 (22.606, 25.908) -> (22.352, 25.908)
  arc A62 (22.352, 25.9461) -> (22.352, 25.8699) centre (22.352, 25.908) ccw
  arc A63 (22.606, 25.8699) -> (22.606, 25.9461) centre (22.606, 25.908) ccw
  line L31 (22.352, 25.908) -> (22.352, 24.892)
  arc A64 (22.3139, 24.892) -> (22.3901, 24.892) centre (22.352, 24.892) ccw
  arc A65 (22.3901, 25.908) -> (22.3139, 25.908) centre (22.352, 25.908) ccw
  line L32 (22.352, 24.892) -> (22.606, 24.892)
  line L33 (12.954, 24.892) -> (13.208, 24.892)
  arc A66 (13.208, 24.8539) -> (13.208, 24.9301) centre (13.208, 24.892) ccw
  arc A67 (12.954, 24.9301) -> (12.954, 24.8539) centre (12.954, 24.892) ccw
  line L34 (20.574, 24.638) -> (20.574, 24.892)
  line L35 (13.208, 24.892) -> (13.208, 25.908)
  arc A68 (13.2461, 25.908) -> (13.1699, 25.908) centre (13.208, 25.908) ccw
  arc A69 (13.1699, 24.892) -> (13.2461, 24.892) centre (13.208, 24.892) ccw
  line L36 (13.208, 25.908) -> (12.954, 25.908)
  arc A70 (12.954, 25.9461) -> (12.954, 25.8699) centre (12.954, 25.908) ccw
  arc A71 (13.208, 25.8699) -> (13.208, 25.9461) centre (13.208, 25.908) ccw
  line L37 (12.954, 25.908) -> (12.954, 26.162)
  arc A72 (12.9921, 26.162) -> (12.9159, 26.162) centre (12.954, 26.162) ccw
  arc A73 (12.9159, 25.908) -> (12.9921, 25.908) centre (12.954, 25.908) ccw
  line L38 (12.954, 26.162) -> (12.446, 26.162)
  arc A74 (12.446, 26.2001) -> (12.446, 26.1239) centre (12.446, 26.162) ccw
  arc A75 (12.954, 26.1239) -> (12.954, 26.2001) centre (12.954, 26.162) ccw
  line L39 (12.446, 26.162) -> (12.446, 25.908)
  arc A76 (12.4079, 25.908) -> (12.4841, 25.908) centre (12.446, 25.908) ccw
  arc A77 (12.4841, 26.162) -> (12.4079, 26.162) centre (12.446, 26.162) ccw
  line L40 (12.446, 25.908) -> (12.192, 25.908)
  arc A78 (12.192, 25.9461) -> (12.192, 25.8699) centre (12.192, 25.908) ccw
  arc A79 (12.446, 25.8699) -> (12.446, 25.9461) centre (12.446, 25.908) ccw
  line L41 (12.192, 25.908) -> (12.192, 24.892)
  arc A80 (12.1539, 24.892) -> (12.2301, 24.892) centre (12.192, 24.892) ccw
  arc A81 (12.2301, 25.908) -> (12.1539, 25.908) centre (12.192, 25.908) ccw
  line L42 (12.192, 24.892) -> (12.446, 24.892)
  arc A82 (12.446, 24.8539) -> (12.446, 24.9301) centre (12.446, 24.892) ccw
  arc A83 (12.192, 24.9301) -> (12.192, 24.8539) centre (12.192, 24.892) ccw
  line L43 (12.446, 24.892) -> (12.446, 24.638)
  arc A84 (12.4079, 24.638) -> (12.4841, 24.638) centre (12.446, 24.638) ccw
  arc A85 (12.4841, 24.892) -> (12.4079, 24.892) centre (12.446, 24.892) ccw
  line L44 (12.446, 24.638) -> (12.954, 24.638)
  arc A86 (12.954, 24.5999) -> (12.954, 24.6761) centre (12.954, 24.638) ccw
  arc A87 (12.446, 24.6761) -> (12.446, 24.5999) centre (12.446, 24.638) ccw
  arc A88 (17.9959, 25.908) -> (18.0721, 25.908) centre (18.034, 25.908) ccw
  line L45 (18.034, 26.162) -> (17.526, 26.162)
  arc A89 (17.526, 26.2001) -> (17.526, 26.1239) centre (17.526, 26.162) ccw
  arc A90 (18.034, 26.1239) -> (18.034, 26.2001) centre (18.034, 26.162) ccw
  line L46 (17.526, 26.162) -> (17.526, 25.908)
  arc A91 (17.4879, 25.908) -> (17.5641, 25.908) centre (17.526, 25.908) ccw
  arc A92 (17.5641, 26.162) -> (17.4879, 26.162) centre (17.526, 26.162) ccw
  line L47 (17.526, 25.908) -> (17.272, 25.908)
  arc A93 (17.272, 25.9461) -> (17.272, 25.8699) centre (17.272, 25.908) ccw
  arc A94 (80.01, 37.0205) -> (80.01, 33.4645) centre (80.01, 35.2425) ccw
  arc A95 (80.01, 33.4645) -> (80.01, 37.0205) centre (80.01, 35.2425) ccw
  arc A96 (74.9808, 37.0205) -> (74.9808, 33.4645) centre (74.9808, 35.2425) ccw
  arc A97 (74.9808, 33.4645) -> (74.9808, 37.0205) centre (74.9808, 35.2425) ccw
  arc A98 (78.9671, 33.8186) -> (79.0209, 33.8724) centre (78.994, 33.8455) ccw
  arc A99 (78.6399, 34.2534) -> (78.5861, 34.1996) centre (78.613, 34.2265) ccw
  line L48 (78.994, 33.8455) -> (78.613, 34.2265)
  arc A100 (81.3801, 36.2316) -> (81.4339, 36.2854) centre (81.407, 36.2585) ccw
  arc A101 (81.0529, 36.6664) -> (80.9991, 36.6126) centre (81.026, 36.6395) ccw
  line L49 (81.407, 36.2585) -> (81.026, 36.6395)
  arc A102 (73.9379, 33.8186) -> (73.9917, 33.8724) centre (73.9648, 33.8455) ccw
  arc A103 (73.6107, 34.2534) -> (73.5569, 34.1996) centre (73.5838, 34.2265) ccw
  line L50 (73.9648, 33.8455) -> (73.5838, 34.2265)
  arc A104 (76.3509, 36.2316) -> (76.4047, 36.2854) centre (76.3778, 36.2585) ccw
  arc A105 (76.0237, 36.6664) -> (75.9699, 36.6126) centre (75.9968, 36.6395) ccw
  line L51 (76.3778, 36.2585) -> (75.9968, 36.6395)
  arc A106 (81.1338, 36.1507) -> (80.9182, 36.3663) centre (81.026, 36.2585) ccw
  arc A107 (78.8862, 34.3343) -> (79.1018, 34.1187) centre (78.994, 34.2265) ccw
  line L52 (81.026, 36.2585) -> (78.994, 34.2265)
  arc A108 (76.1046, 36.1507) -> (75.889, 36.3663) centre (75.9968, 36.2585) ccw
  arc A109 (73.857, 34.3343) -> (74.0726, 34.1187) centre (73.9648, 34.2265) ccw
  line L53 (75.9968, 36.2585) -> (73.9648, 34.2265)
  arc A110 (81.0529, 36.6126) -> (80.9991, 36.6664) centre (81.026, 36.6395) ccw
  arc A111 (78.5861, 34.2534) -> (78.6399, 34.1996) centre (78.613, 34.2265) ccw
  line L54 (81.026, 36.6395) -> (78.613, 34.2265)
  arc A112 (81.4339, 36.2316) -> (81.3801, 36.2854) centre (81.407, 36.2585) ccw
  arc A113 (78.9671, 33.8724) -> (79.0209, 33.8186) centre (78.994, 33.8455) ccw
  line L55 (81.407, 36.2585) -> (78.994, 33.8455)
  arc A114 (76.4047, 36.2316) -> (76.3509, 36.2854) centre (76.3778, 36.2585) ccw
  arc A115 (73.9379, 33.8724) -> (73.9917, 33.8186) centre (73.9648, 33.8455) ccw
  line L56 (76.3778, 36.2585) -> (73.9648, 33.8455)
  arc A116 (76.0237, 36.6126) -> (75.9699, 36.6664) centre (75.9968, 36.6395) ccw
  arc A117 (73.5569, 34.2534) -> (73.6107, 34.1996) centre (73.5838, 34.2265) ccw
  line L57 (75.9968, 36.6395) -> (73.5838, 34.2265)
  arc A118 (22.5679, 24.638) -> (22.6441, 24.638) centre (22.606, 24.638) ccw
  line L58 (22.606, 24.892) -> (22.606, 24.638)
  arc A119 (22.352, 24.9301) -> (22.352, 24.8539) centre (22.352, 24.892) ccw
  arc A120 (17.526, 25.8699) -> (17.526, 25.9461) centre (17.526, 25.908) ccw
  line L59 (17.272, 25.908) -> (17.272, 24.892)
  arc A121 (17.2339, 24.892) -> (17.3101, 24.892) centre (17.272, 24.892) ccw
  arc A122 (17.3101, 25.908) -> (17.2339, 25.908) centre (17.272, 25.908) ccw
  line L60 (17.272, 24.892) -> (17.526, 24.892)
  arc A123 (17.526, 24.8539) -> (17.526, 24.9301) centre (17.526, 24.892) ccw
  arc A124 (22.606, 24.6761) -> (22.606, 24.5999) centre (22.606, 24.638) ccw
  arc A125 (17.272, 24.9301) -> (17.272, 24.8539) centre (17.272, 24.892) ccw
  line L61 (17.526, 24.892) -> (17.526, 24.638)
  arc A126 (23.114, 24.5999) -> (23.114, 24.6761) centre (23.114, 24.638) ccw
  arc A127 (17.4879, 24.638) -> (17.5641, 24.638) centre (17.526, 24.638) ccw
  arc A128 (17.5641, 24.892) -> (17.4879, 24.892) centre (17.526, 24.892) ccw
  line L62 (17.526, 24.638) -> (18.034, 24.638)
  line L63 (20.828, 24.892) -> (20.828, 25.908)
  arc A129 (18.034, 24.5999) -> (18.034, 24.6761) centre (18.034, 24.638) ccw
  arc A130 (17.526, 24.6761) -> (17.526, 24.5999) centre (17.526, 24.638) ccw
  line L64 (15.494, 24.638) -> (15.494, 24.892)
  line L65 (22.606, 24.638) -> (23.114, 24.638)
  arc A131 (15.5321, 24.892) -> (15.4559, 24.892) centre (15.494, 24.892) ccw
  arc A132 (15.4559, 24.638) -> (15.5321, 24.638) centre (15.494, 24.638) ccw
  line L66 (15.494, 24.892) -> (15.748, 24.892)
  arc A133 (15.748, 24.8539) -> (15.748, 24.9301) centre (15.748, 24.892) ccw
  arc A134 (15.494, 24.9301) -> (15.494, 24.8539) centre (15.494, 24.892) ccw
  line L67 (15.748, 24.892) -> (15.748, 25.908)
  arc A135 (15.7861, 25.908) -> (15.7099, 25.908) centre (15.748, 25.908) ccw
  arc A136 (15.7099, 24.892) -> (15.7861, 24.892) centre (15.748, 24.892) ccw
  line L68 (45.847, 26.162) -> (45.847, 25.908)
  arc A137 (45.8089, 25.908) -> (45.8851, 25.908) centre (45.847, 25.908) ccw
  arc A138 (45.8851, 26.162) -> (45.8089, 26.162) centre (45.847, 26.162) ccw
  line L69 (45.847, 25.908) -> (45.593, 25.908)
  arc A139 (20.7899, 24.892) -> (20.8661, 24.892) centre (20.828, 24.892) ccw
  arc A140 (45.593, 25.9461) -> (45.593, 25.8699) centre (45.593, 25.908) ccw
  arc A141 (45.847, 25.8699) -> (45.847, 25.9461) centre (45.847, 25.908) ccw
  line L70 (45.593, 25.908) -> (45.593, 24.892)
  arc A142 (45.5549, 24.892) -> (45.6311, 24.892) centre (45.593, 24.892) ccw
  arc A143 (45.6311, 25.908) -> (45.5549, 25.908) centre (45.593, 25.908) ccw
  line L71 (45.593, 24.892) -> (45.847, 24.892)
  arc A144 (45.847, 24.8539) -> (45.847, 24.9301) centre (45.847, 24.892) ccw
  arc A145 (45.593, 24.9301) -> (45.593, 24.8539) centre (45.593, 24.892) ccw
  line L72 (45.847, 24.892) -> (45.847, 24.638)
  arc A146 (45.8089, 24.638) -> (45.8851, 24.638) centre (45.847, 24.638) ccw
  arc A147 (45.8851, 24.892) -> (45.8089, 24.892) centre (45.847, 24.892) ccw
  line L73 (45.847, 24.638) -> (46.355, 24.638)
  arc A148 (46.355, 24.5999) -> (46.355, 24.6761) centre (46.355, 24.638) ccw
  arc A149 (45.847, 24.6761) -> (45.847, 24.5999) centre (45.847, 24.638) ccw
  line L74 (46.355, 24.638) -> (46.355, 24.892)
  arc A150 (46.3931, 24.892) -> (46.3169, 24.892) centre (46.355, 24.892) ccw
  arc A151 (46.3169, 24.638) -> (46.3931, 24.638) centre (46.355, 24.638) ccw
  line L75 (46.355, 24.892) -> (46.609, 24.892)
  arc A152 (46.609, 24.8539) -> (46.609, 24.9301) centre (46.609, 24.892) ccw
  arc A153 (46.355, 24.9301) -> (46.355, 24.8539) centre (46.355, 24.892) ccw
  line L76 (46.609, 24.892) -> (46.609, 25.908)
  arc A154 (46.6471, 25.908) -> (46.5709, 25.908) centre (46.609, 25.908) ccw
  arc A155 (46.5709, 24.892) -> (46.6471, 24.892) centre (46.609, 24.892) ccw
  line L77 (46.609, 25.908) -> (46.355, 25.908)
  arc A156 (46.355, 25.9461) -> (46.355, 25.8699) centre (46.355, 25.908) ccw
  arc A157 (46.609, 25.8699) -> (46.609, 25.9461) centre (46.609, 25.908) ccw
  line L78 (46.355, 25.908) -> (46.355, 26.162)
  arc A158 (46.3931, 26.162) -> (46.3169, 26.162) centre (46.355, 26.162) ccw
  arc A159 (46.3169, 25.908) -> (46.3931, 25.908) centre (46.355, 25.908) ccw
  line L79 (46.355, 26.162) -> (45.847, 26.162)
  arc A160 (45.847, 26.2001) -> (45.847, 26.1239) centre (45.847, 26.162) ccw
  arc A161 (46.355, 26.1239) -> (46.355, 26.2001) centre (46.355, 26.162) ccw
  line L80 (48.387, 26.162) -> (48.387, 25.908)
  arc A162 (48.3489, 25.908) -> (48.4251, 25.908) centre (48.387, 25.908) ccw
  arc A163 (48.4251, 26.162) -> (48.3489, 26.162) centre (48.387, 26.162) ccw
  line L81 (48.387, 25.908) -> (48.133, 25.908)
  arc A164 (48.133, 25.9461) -> (48.133, 25.8699) centre (48.133, 25.908) ccw
  arc A165 (48.387, 25.8699) -> (48.387, 25.9461) centre (48.387, 25.908) ccw
  line L82 (48.133, 25.908) -> (48.133, 24.892)
  arc A166 (48.0949, 24.892) -> (48.1711, 24.892) centre (48.133, 24.892) ccw
  arc A167 (48.1711, 25.908) -> (48.0949, 25.908) centre (48.133, 25.908) ccw
  line L83 (48.133, 24.892) -> (48.387, 24.892)
  arc A168 (20.574, 24.9301) -> (20.574, 24.8539) centre (20.574, 24.892) ccw
  arc A169 (48.387, 24.8539) -> (48.387, 24.9301) centre (48.387, 24.892) ccw
  arc A170 (48.133, 24.9301) -> (48.133, 24.8539) centre (48.133, 24.892) ccw
  line L84 (48.387, 24.892) -> (48.387, 24.638)
  arc A171 (48.3489, 24.638) -> (48.4251, 24.638) centre (48.387, 24.638) ccw
  arc A172 (22.606, 24.8539) -> (22.606, 24.9301) centre (22.606, 24.892) ccw
  arc A173 (48.4251, 24.892) -> (48.3489, 24.892) centre (48.387, 24.892) ccw
  line L85 (48.387, 24.638) -> (48.895, 24.638)
  arc A174 (48.895, 24.5999) -> (48.895, 24.6761) centre (48.895, 24.638) ccw
  arc A175 (48.387, 24.6761) -> (48.387, 24.5999) centre (48.387, 24.638) ccw
  line L86 (48.895, 24.638) -> (48.895, 24.892)
  arc A176 (48.9331, 24.892) -> (48.8569, 24.892) centre (48.895, 24.892) ccw
  arc A177 (48.8569, 24.638) -> (48.9331, 24.638) centre (48.895, 24.638) ccw
  line L87 (48.895, 24.892) -> (49.149, 24.892)
  arc A178 (49.149, 24.8539) -> (49.149, 24.9301) centre (49.149, 24.892) ccw
  arc A179 (48.895, 24.9301) -> (48.895, 24.8539) centre (48.895, 24.892) ccw
  line L88 (49.149, 24.892) -> (49.149, 25.908)
  arc A180 (49.1871, 25.908) -> (49.1109, 25.908) centre (49.149, 25.908) ccw
  arc A181 (49.1109, 24.892) -> (49.1871, 24.892) centre (49.149, 24.892) ccw
  line L89 (49.149, 25.908) -> (48.895, 25.908)
  arc A182 (48.895, 25.9461) -> (48.895, 25.8699) centre (48.895, 25.908) ccw
  arc A183 (49.149, 25.8699) -> (49.149, 25.9461) centre (49.149, 25.908) ccw
  line L90 (48.895, 25.908) -> (48.895, 26.162)
  arc A184 (48.9331, 26.162) -> (48.8569, 26.162) centre (48.895, 26.162) ccw
  arc A185 (48.8569, 25.908) -> (48.9331, 25.908) centre (48.895, 25.908) ccw
  line L91 (48.895, 26.162) -> (48.387, 26.162)
  arc A186 (48.387, 26.2001) -> (48.387, 26.1239) centre (48.387, 26.162) ccw
  arc A187 (48.895, 26.1239) -> (48.895, 26.2001) centre (48.895, 26.162) ccw
  line L92 (50.927, 26.162) -> (50.927, 25.908)
  arc A188 (50.8889, 25.908) -> (50.9651, 25.908) centre (50.927, 25.908) ccw
  arc A189 (50.9651, 26.162) -> (50.8889, 26.162) centre (50.927, 26.162) ccw
  line L93 (50.927, 25.908) -> (50.673, 25.908)
  arc A190 (50.673, 25.9461) -> (50.673, 25.8699) centre (50.673, 25.908) ccw
  arc A191 (50.927, 25.8699) -> (50.927, 25.9461) centre (50.927, 25.908) ccw
  line L94 (50.673, 25.908) -> (50.673, 24.892)
  arc A192 (50.6349, 24.892) -> (50.7111, 24.892) centre (50.673, 24.892) ccw
  arc A193 (50.7111, 25.908) -> (50.6349, 25.908) centre (50.673, 25.908) ccw
  line L95 (50.673, 24.892) -> (50.927, 24.892)
  arc A194 (50.927, 24.8539) -> (50.927, 24.9301) centre (50.927, 24.892) ccw
  arc A195 (50.673, 24.9301) -> (50.673, 24.8539) centre (50.673, 24.892) ccw
  line L96 (50.927, 24.892) -> (50.927, 24.638)
  arc A196 (50.8889, 24.638) -> (50.9651, 24.638) centre (50.927, 24.638) ccw
  arc A197 (50.9651, 24.892) -> (50.8889, 24.892) centre (50.927, 24.892) ccw
  line L97 (50.927, 24.638) -> (51.435, 24.638)
  arc A198 (51.435, 24.5999) -> (51.435, 24.6761) centre (51.435, 24.638) ccw
  arc A199 (50.927, 24.6761) -> (50.927, 24.5999) centre (50.927, 24.638) ccw
  line L98 (51.435, 24.638) -> (51.435, 24.892)
  arc A200 (51.4731, 24.892) -> (51.3969, 24.892) centre (51.435, 24.892) ccw
  arc A201 (51.3969, 24.638) -> (51.4731, 24.638) centre (51.435, 24.638) ccw
  line L99 (51.435, 24.892) -> (51.689, 24.892)
  arc A202 (20.828, 24.8539) -> (20.828, 24.9301) centre (20.828, 24.892) ccw
  arc A203 (51.689, 24.8539) -> (51.689, 24.9301) centre (51.689, 24.892) ccw
  arc A204 (51.435, 24.9301) -> (51.435, 24.8539) centre (51.435, 24.892) ccw
  line L100 (51.689, 24.892) -> (51.689, 25.908)
  arc A205 (51.7271, 25.908) -> (51.6509, 25.908) centre (51.689, 25.908) ccw
  arc A206 (51.6509, 24.892) -> (51.7271, 24.892) centre (51.689, 24.892) ccw
  line L101 (51.689, 25.908) -> (51.435, 25.908)
  arc A207 (51.435, 25.9461) -> (51.435, 25.8699) centre (51.435, 25.908) ccw
  arc A208 (51.689, 25.8699) -> (51.689, 25.9461) centre (51.689, 25.908) ccw
  line L102 (51.435, 25.908) -> (51.435, 26.162)
  arc A209 (51.4731, 26.162) -> (51.3969, 26.162) centre (51.435, 26.162) ccw
  arc A210 (51.3969, 25.908) -> (51.4731, 25.908) centre (51.435, 25.908) ccw
  line L103 (51.435, 26.162) -> (50.927, 26.162)